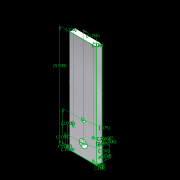
# Autodesk Inventor part: xtower1
Saved by Autodesk Inventor 2012 (Build 160160000, 160)
## iProperties
Created: 2011-09-19
Part Number: xtower1
Material: Default
Document SubType Name: Modeling
Designer: shane
Density: 1 g/cm^3
Author: shane
Autodesk Inventor part; units mm, degrees
ref_plane "YZ Plane" through (0, 0, 0) normal (1, 0, 0) x (0, 1, 0)
ref_plane "XZ Plane" through (0, 0, 0) normal (0, 1, 0) x (-1, 0, 0)
ref_plane "XY Plane" through (0, 0, 0) normal (0, 0, 1) x (1, 0, 0)
sketch "Sketch1" plane through (0, 0, 0) normal (0, 0, 1) x (1, 0, 0)
  line L0 (0, -139.3108) -> (63.5, -139.3108)
  line L1 (63.5, -139.3108) -> (63.5, 101.9892)
  line L2 (63.5, 101.9892) -> (0, 101.9892)
  line L3 (0, 101.9892) -> (0, -139.3108)
  point P0 (0, 0)
  dimension "d0" = 63.5
  dimension "d1" = 241.3
  constraints: 8 end point, 2 parallel, 1 horizontal, 1 perpendicular
  measures "d0" distance of L2.end L1.end
  measures "d1" distance of L1.end L0.end
extrude "Extrusion1" add sketch "Sketch1" along normal blind 12.7
hole "Hole15" at (8.128, -134.3578, 12.7) direction (0, 0, -1) diameter 5.08 end through all
hole "Hole16" at (55.372, -134.3578, 12.7) direction (0, 0, -1) diameter 5.08 end through all
hole "Hole17" at (8.128, -87.1138, 12.7) direction (0, 0, -1) diameter 5.08 end through all
hole "Hole18" at (55.372, -87.1138, 12.7) direction (0, 0, -1) diameter 5.08 end through all
hole "Hole19" at (31.75, -63.1108, 12.7) direction (0, 0, -1) diameter 9.525 end through all
hole "Hole20" at (31.75, -110.7358, 12.7) direction (0, 0, -1) diameter 19.05 end through all
sketch "Font" plane through (0, 0, 12.7) normal (0, 0, 1) x (1, 0, 0)
  circle A0 centre (31.75, -110.7358) radius 9.525 projected
  circle A1 centre (31.75, -63.1108) radius 4.7625 projected
  circle A2 centre (55.372, -87.1138) radius 2.54 projected
  circle A3 centre (8.128, -87.1138) radius 2.54 projected
  circle A4 centre (55.372, -134.3578) radius 2.54 projected
  circle A5 centre (8.128, -134.3578) radius 2.54 projected
  line L0 (0, -139.3108) -> (0, 101.9892) projected
  line L1 (63.5, -139.3108) -> (0, -139.3108) projected
  line L2 (63.5, 101.9892) -> (63.5, -139.3108) projected
  line L3 (0, 101.9892) -> (63.5, 101.9892) projected
  point P0 (0, 0)
  dimension "d220" = 241.3
  dimension "d221" = 5.08
  dimension "d222" = 9.525
  dimension "d223" = 19.05
  dimension "d224" = 8.128
  dimension "d225" = 4.953
  dimension "d226" = 28.575
  dimension "d227" = 76.2
  dimension "d228" = 8.128
  dimension "d229" = 4.953
  dimension "d230" = 52.197
  dimension "d231" = 52.197
  dimension "d238" = 31.75
  measures "d220" distance of L0.start L0.end
  measures "d221" diameter of A2
  measures "d222" diameter of A1
  measures "d223" diameter of A0
  measures "d224" distance from line of A3.centre L0
  measures "d225" distance from line of A5.centre L1
  measures "d226" distance from line of A0.centre L1
  measures "d227" distance from line of L1 A1.centre
  measures "d228" distance from line of A2.centre L2
  measures "d229" distance from line of L1 A4.centre
  measures "d230" distance from line of A3.centre L1
  measures "d231" distance from line of A2.centre L1
  measures "d238" distance from line of L2 A0.centre
sketch "bottom" plane through (0, -139.3108, 0) normal (0, -1, 0) x (1, 0, 0)
  line L0 (63.5, 12.7) -> (0, 12.7) projected
  line L1 (0, 0) -> (0, 12.7) projected
  line L2 (0, 0) -> (63.5, 0) projected
  line L3 (63.5, 0) -> (63.5, 12.7) projected
  point P0 (47.752, 6.35)
  point P1 (15.748, 6.35)
  dimension "d233" = 12.7
  measures "d233" distance of L2.end L0.start
sketch "Right" plane through (63.5, -139.3108, 0) normal (1, 0, 0) x (0, 0, -1)
  line L0 (-12.7, 241.3) -> (-12.7, 0) projected
  line L1 (0, 0) -> (-12.7, 0) projected
  line L2 (0, 0) -> (0, 241.3) projected
  line L3 (0, 241.3) -> (-12.7, 241.3) projected
  point P0 (0, 139.3108)
hole "Hole25" at (63.5, -126.6108, 6.35) direction (-1, 0, 0) diameter 4.826 depth 19.05 tip angle 118
hole "Hole26" at (63.5, -101.2108, 6.35) direction (-1, 0, 0) diameter 4.826 depth 19.05 tip angle 118
sketch "Sketch6" plane through (63.5, -139.3108, 0) normal (1, 0, 0) x (0, 0, -1)
  circle A0 centre (-6.35, 38.1) radius 2.413 projected
  circle A1 centre (-6.35, 12.7) radius 2.413 projected
  line L0 (-12.7, 241.3) -> (-12.7, 0) projected
  line L1 (0, 0) -> (-12.7, 0) projected
  line L2 (0, 0) -> (0, 241.3) projected
  line L3 (0, 241.3) -> (-12.7, 241.3) projected
  point P0 (0, 139.3108)
  dimension "d257" = 4.826
  dimension "d260" = 38.1
  dimension "d261" = 12.7
  measures "d257" diameter of A0
  measures "d260" distance from line of L1 A0.centre
  measures "d261" distance from line of L1 A1.centre
body "Solid1"
